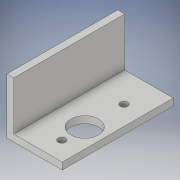
# Autodesk Inventor part: 2in L-Bracket
Saved by Autodesk Inventor 2018 (Build 220112000, 112)
## iProperties
Created: 2020-01-24
Part Number: 2in L-Bracket
Material: Generic
Document SubType Name: Modeling
Designer: S-2512711
Density: 1 g/cm^3
Appearance: Default
Author: S-2512711
Autodesk Inventor part; units mm, degrees
ref_plane "YZ Plane" through (0, 0, 0) normal (1, 0, 0) x (0, 1, 0)
ref_plane "XZ Plane" through (0, 0, 0) normal (0, 1, 0) x (-1, 0, 0)
ref_plane "XY Plane" through (0, 0, 0) normal (0, 0, 1) x (1, 0, 0)
sketch "Sketch1" plane through (0, 0, 0) normal (0, 0, 1) x (1, 0, 0)
  line L0 (0, 0) -> (3.175, 0)
  line L1 (3.175, 0) -> (3.175, 25.4)
  line L2 (3.175, 25.4) -> (0, 25.4)
  line L3 (0, 25.4) -> (0, 0)
  line L4 (0, 0) -> (25.4, 0)
  line L5 (25.4, 0) -> (25.4, 3.175)
  line L6 (25.4, 3.175) -> (0, 3.175)
  line L7 (0, 3.175) -> (0, 0)
  dimension "d0" = 3.175
  dimension "d1" = 25.4
  dimension "d2" = 25.4
  dimension "d3" = 3.175
  constraints: 16 end point, 4 parallel, 2 horizontal, 2 perpendicular
  measures "d0" distance of L2.end L1.end
  measures "d1" distance of L1.end L0.end
  measures "d2" distance of L6.end L5.end
  measures "d3" distance of L5.end L4.end
extrude "Extrusion1" add sketch "Sketch1" along normal blind 50.8
sketch "Sketch2" plane through (3.175, 3.175, 0) normal (0, 1, 0) x (1, 0, 0)
  line L0 (-3.175, -50.8) -> (22.225, -50.8) construction
  line L1 (-3.175, -50.8) -> (13.462, -50.8) construction
  line L2 (13.462, -50.8) -> (13.462, -31.75) construction
  line L3 (13.462, -50.8) -> (32.512, -50.8) construction
  circle A0 centre (13.462, -31.75) radius 6.35
  point P0 (-3.175, 0)
  dimension "d6" = 16.637
  dimension "d7" = 19.05
  dimension "d8" = 90
  dimension "d9" = 12.7
  constraints: 6 end point, 1 centre point, 1 coincident, 1 horizontal, 1 perpendicular, 1 point on line, 1 vertical
  measures "d6" distance of L0.start L1.end
  measures "d7" distance of L1.end L2.end
  measures "d8" angle of L3 L2
  measures "d9" diameter of A0
extrude "Extrusion2" cut sketch "Sketch2" against normal blind 50.8
sketch "Sketch3" plane through (3.175, 3.175, 0) normal (0, 1, 0) x (1, 0, 0)
  circle A0 centre (13.462, -31.75) radius 6.35 construction
  line L0 (13.462, -31.75) -> (13.462, -42.2402) construction
  line L1 (13.462, -42.2402) -> (13.462, -13.7414) construction
  circle A1 centre (13.462, -42.2402) radius 1.7018
  circle A2 centre (13.462, -13.7414) radius 1.7018
  point P0 (-3.175, 0)
  dimension "d12" = 10.4902
  dimension "d13" = 28.4988
  dimension "d14" = 3.4036
  dimension "d15" = 3.4036
  constraints: 4 end point, 2 centre point, 2 coincident, 1 point on line, 1 vertical
  measures "d12" distance of L0.start L0.end
  measures "d13" distance of L0.end L1.end
  measures "d14" diameter of A1
  measures "d15" diameter of A2
extrude "Extrusion3" cut sketch "Sketch3" against normal blind 50.8
body "Solid1"
